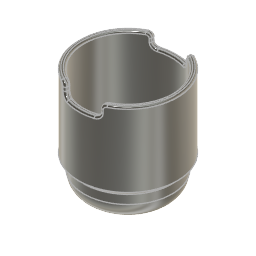
basic_self_watering_potjie_finger_cutouts (Autodesk Fusion 360 design; units mm, degrees)
Autodesk Fusion 360 part; units mm, degrees
sketch "simple_potjie_base" plane through (0, 0, 0) normal (0, 0, 1) x (1, 0, 0)
  circle A0 centre (0, 0) radius 25
  circle A1 centre (0, 0) radius 28
  circle A2 centre (0, 0) radius 21.75
  line L0 (0, 0) -> (-7, 0)
  line L1 (0, 0) -> (7, 0)
  circle A3 centre (7, 0) radius 4
  circle A4 centre (-7, 0) radius 4
  dimension "d4" = 50
  dimension "d5" = 56
  dimension "d36" = 43.5
  dimension "d46" = 7
  dimension "d47" = 7
  dimension "d48" = 8
  dimension "d49" = 8
  constraint coincident A0.centre A1.centre
  constraint concentric A1 A2
  constraint horizontal L0
  constraint parallel L0 L1
  constraint coincident L1.end A3.centre
  constraint coincident L0.end A4.centre
  measures "d4" diameter of A0
  measures "d5" diameter of A1
  measures "d36" diameter of A2
  measures "d46" distance of A0.centre L0.end
  measures "d47" distance of A0.centre L1.end
  measures "d48" diameter of A3
  measures "d49" diameter of A4
sketch "finger_cutouts" plane through (0, 0, 0) normal (0, 1, 0) x (1, 0, 0)
  line L0 (0, 0) -> (0, -60)
  line L1 (0, -60) -> (10, -60)
  line L2 (10, -60) -> (-10, -60)
  line L3 (-10, -60) -> (-10, -53)
  line L4 (-10, -53) -> (10, -53)
  line L5 (10, -53) -> (10, -60)
  dimension "d18" = 60
  dimension "d20" = 10
  dimension "d21" = 20
  dimension "d22" = 7
  constraint coincident L0.start origin
  constraint vertical L0
  constraint perpendicular L0 L1
  constraint horizontal L2
  constraint vertical L3
  constraint horizontal L4
  constraint vertical L5
  measures "d18" distance of L0.start L0.end
  measures "d20" distance of L0.end L1.end
  measures "d21" distance of L1.end L2.end
  measures "d22" distance of L1.end L4.end
extrude "Extrude1" add sketch "simple_potjie_base" along normal blind 3 contours A0 | A2 | A3 | A4 makes body 1
extrude "Extrude2" add sketch "simple_potjie_base" along normal blind 60 and the other way blind -15 separate body contours A1 makes body 2
chamfer "Chamfer2" distance 3 angle 45 1 edges at (-23.3082, -9.0404, 3) on bodies 1
extrude "Extrude4" add sketch "simple_potjie_base" along normal blind 18 contours A0 bodies 1 2
chamfer "Chamfer3" distance 3 angle 45 1 edges at (-26.1052, -10.1252, 15) on bodies 1 2
chamfer "Chamfer4" distance 3 angle 45 1 edges at (-23.3082, 9.0404, 18) on bodies 1
fillet "Fillet5" radius 7 1 edges at (-20.2781, -7.8651, 3) on bodies 1
fillet "Fillet6" radius 10 1 edges at (-23.3082, -9.0404, 0) on bodies 1
extrude "Extrude5" cut sketch "simple_potjie_base" along normal blind 3 contours A3 | A4 bodies 1
extrude "Extrude6" cut sketch "finger_cutouts" along normal blind 28 bodies 1
fillet "Fillet9" radius 2.5 2 edges at (-10, 24.5331, 53) (10, 24.5331, 53) on bodies 1
fillet "Fillet10" radius 2.5 2 edges at (-10, 24.5331, 60) (10, 24.5331, 60) on bodies 1
pattern_circular "C-Pattern2" count 2 over 360 about axis through (0, 0, 0) along (0, 0, 1) of "Extrude6", "Fillet9", "Fillet10"
fillet "Fillet12" radius 1 32 edges at (10, -22.9129, 56.5) (9.2477, -23.2267, 53.7124) (0, -25, 53) (-9.2477, -23.2267, 53.7124) (-10, -22.9129, 56.5) (-10.7866, -22.5532, 59.3203) (-25, 0, 60) (-10.7866, 22.5532, 59.3203) (-10, 22.9129, 56.5) (-9.2477, 23.2267, 53.7124) (0, 25, 53) (9.2477, 23.2267, 53.7124) (10, 22.9129, 56.5) (10.7866, 22.5532, 59.3203) (25, 0, 60) (10.7866, -22.5532, 59.3203) (10, 26.1534, 56.5) (9.2519, 26.4273, 53.7165) (0, 28, 53) (-9.2519, 26.4273, 53.7165) (-10, 26.1534, 56.5) (-10.774, 25.8442, 59.3084) (-28, 0, 60) (-10.774, -25.8442, 59.3084) (-10, -26.1534, 56.5) (-9.2519, -26.4273, 53.7165) (0, -28, 53) (9.2519, -26.4273, 53.7165) (10, -26.1534, 56.5) (10.774, -25.8442, 59.3084) (28, 0, 60) (10.774, 25.8442, 59.3084) on bodies 1
equation "wall_thinkness = 3 mm" comment "Thickness of the walls of the entire print."
equation "pot_height = 60 mm" comment "Total height of the pot. Including the narrowing insert part."
equation "pot_inner_diameter = 50 mm" comment "Inner diameter of the upper part of the pot."
equation "d4 = pot_inner_diameter"
equation "d5 = pot_inner_diameter + ( 2 * wall_thinkness )"
equation "d6 = wall_thinkness"
equation "d8 = pot_height"
equation "pot_bottom_fillet = 10 mm" comment "Fillet/Rounding of the bottom of the pot. Inner fillet calculated automatically."
equation "pot_finger_cutout_num = 2" comment "Number of finger cutouts around the upper brim."
equation "pot_finger_cutout_width = 20 mm" comment "Width of the finger cutout."
equation "d18 = pot_height"
equation "pot_finger_cutout_height = 7 mm" comment "Height of the finger cutout."
equation "d20 = pot_finger_cutout_width / 2"
equation "d21 = pot_finger_cutout_width"
equation "d22 = pot_finger_cutout_height"
equation "d31 = wall_thinkness"
equation "d32 = wall_thinkness"
equation "d33 = -pot_bottom_insert_height"
equation "pot_bottom_insert_height = 15 mm" comment "The height of the bottom narrower portion that will fit into the lower pot."
equation "d36 = pot_inner_diameter - ( 2 * wall_thinkness ) - 0.5 mm"
equation "d37 = pot_bottom_insert_height + wall_thinkness"
equation "d39 = wall_thinkness"
equation "d41 = pot_bottom_fillet - wall_thinkness"
equation "d43 = pot_bottom_fillet"
equation "wick_holes_distance_apart = 6 mm" comment "Distance between the holes for the wick to go through."
equation "wick_hole_diameter = 8 mm" comment "Diameter of the holes for the wick to go through."
equation "d46 = wick_holes_distance_apart / 2 + wick_hole_diameter / 2"
equation "d47 = wick_holes_distance_apart / 2 + wick_hole_diameter / 2"
equation "d48 = wick_hole_diameter"
equation "d49 = wick_hole_diameter"
equation "d50 = wall_thinkness"
equation "d56 = pot_inner_diameter / 2 + wall_thinkness"
equation "d59 = pot_finger_cutout_height / 2 - 1 mm"
equation "d61 = pot_finger_cutout_height / 2 - 1 mm"
equation "d64 = pot_finger_cutout_num"
named bodies: "simple_potjie"
